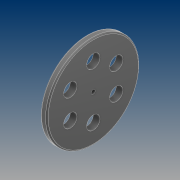
# Autodesk Inventor part: 05_Banh_xe
Saved by Autodesk Inventor 2021 (Build 250183000, 183)
## iProperties
Created: 2024-03-25
Part Number: 05_Banh_xe
Material: Acetal Resin, Black
Document SubType Name: Modeling
Designer: Admin
Density: 1.425 g/cm^3
Appearance: Smooth - Black
Author: Admin
Autodesk Inventor part; units mm, degrees
ref_plane "YZ Plane" through (0, 0, 0) normal (1, 0, 0) x (0, 1, 0)
ref_plane "XZ Plane" through (0, 0, 0) normal (0, 1, 0) x (-1, 0, 0)
ref_plane "XY Plane" through (0, 0, 0) normal (0, 0, 1) x (1, 0, 0)
sketch "Sketch1" plane through (0, 0, 0) normal (1, 0, 0) x (0, 1, 0)
  circle A0 centre (0, 0) radius 3
  circle A1 centre (0, 0) radius 70
  dimension "d0" = 140
  dimension "d1" = 6
  constraints: 2 centre point, 2 coincident
  measures "d0" diameter of A1
  measures "d1" diameter of A0
extrude "Extrusion1" add sketch "Sketch1" along normal blind 10
fillet "Fillet1" radius 2 2 edges at (10, -70, 0) (0, -70, 0)
sketch "Sketch2" plane through (10, 0, 0) normal (1, 0, 0) x (0, 0, -1)
  circle A0 centre (0, 40) radius 10
  circle A1 centre (0, 0) radius 3 projected
  dimension "d5" = 20
  dimension "d6" = 40
  constraints: 1 centre point
  measures "d5" diameter of A0
  measures "d6" distance of A1.centre A0.centre
extrude "Extrusion2" cut sketch "Sketch2" against normal blind 10 contours A0
pattern_circular "Circular Pattern1" count 6 over 360 about axis through (0, 0, 0) along (1, 0, 0) of "Extrusion2"
body "Solid1"
